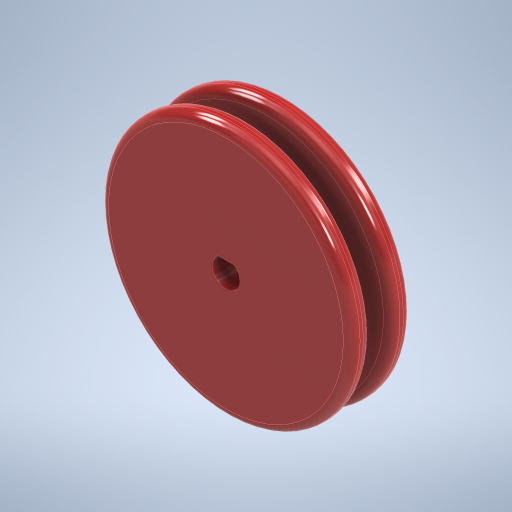
# Autodesk Inventor part: Motor Spool For Door Opener Without Set Screw
Saved by Autodesk Inventor 2024 (Build 280153000, 153)
## iProperties
Created: 2024-01-28
Part Number: Motor Spool For Door Opener Without Set Screw
Material: ABS Plastic
Document SubType Name: Modeling
Designer: himmelb
Density: 1.06 g/cm^3
Appearance: Red
Author: himmelb
Autodesk Inventor part; units mm, degrees
ref_plane "YZ Plane" through (0, 0, 0) normal (1, 0, 0) x (0, 1, 0)
ref_plane "XZ Plane" through (0, 0, 0) normal (0, 1, 0) x (-1, 0, 0)
ref_plane "XY Plane" through (0, 0, 0) normal (0, 0, 1) x (1, 0, 0)
sketch "Sketch1" plane through (0, 0, 0) normal (0, 0, 1) x (1, 0, 0)
  circle A0 centre (0, 0) radius 22.5
  dimension "d0" = 45
  constraints: 1 centre point, 1 coincident
  measures "d0" diameter of A0
extrude "Extrusion1" add sketch "Sketch1" against normal blind 3.5833
sketch "Sketch2" plane through (0, 0, -3.5833) normal (0, 0, -1) x (-1, 0, 0)
  circle A0 centre (0, 0) radius 10
  dimension "d14" = 20
  constraints: 1 centre point
  measures "d14" diameter of A0
extrude "Extrusion2" add sketch "Sketch2" along normal blind 3.5833
sketch "Sketch3" plane through (0, 0, -7.1666) normal (0, 0, -1) x (-1, 0, 0)
  circle A0 centre (0, 0) radius 22.5
  dimension "d19" = 45
  constraints: 1 centre point, 1 coincident
  measures "d19" diameter of A0
extrude "Extrusion3" add sketch "Sketch3" along normal blind 3.5833
fillet "Fillet2" radius 1.5 6 edges at (-22.5, 0, 0) (22.5, 0, -7.1666) (22.5, 0, -10.7499) (-22.5, 0, -3.5833) (10, 0, -7.1666) (10, 0, -3.5833)
sketch "Sketch4" plane through (0, 0, 0) normal (0, 0, 1) x (1, 0, 0)
  arc A0 (-1.5033, 2.01) -> (1.5033, 2.01) centre (0, 0) ccw
  line L0 (-1.5033, 2.01) -> (1.5033, 2.01)
  dimension "d15" = 5.02
  constraints: 2 end point, 2 point on circle, 1 centre point, 1 coincident, 1 horizontal
  measures "d15" diameter of A0
extrude "Extrusion4" cut sketch "Sketch4" against normal through all
body "Solid1"
